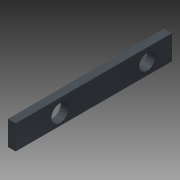
# Autodesk Inventor part: connector
Saved by Autodesk Inventor 2015 (Build 190159000, 159)
## iProperties
Created: 2020-01-20
Part Number: connector
Material: Iron, Cast
Document SubType Name: Modeling
Designer: hp
Density: 7.15 g/cm^3
Appearance: Iron Gray
Author: hp
Autodesk Inventor part; units mm, degrees
ref_plane "YZ Plane" through (0, 0, 0) normal (1, 0, 0) x (0, 1, 0)
ref_plane "XZ Plane" through (0, 0, 0) normal (0, 1, 0) x (-1, 0, 0)
ref_plane "XY Plane" through (0, 0, 0) normal (0, 0, 1) x (1, 0, 0)
sketch "Sketch1" plane through (0, 0, 0) normal (1, 0, 0) x (0, 1, 0)
  line L0 (-28.0063, 19.8873) -> (-28.0062, -488.1127)
  line L1 (-106.9702, 19.8873) -> (-28.0063, 19.8873)
  circle A0 centre (-68.4003, -407.0636) radius 25.4
  line L2 (-106.9702, -488.1127) -> (-28.0062, -488.1127)
  line L3 (-106.9702, -488.1127) -> (-106.9702, 19.8873)
  line L4 (-68.4003, -407.0636) -> (-65.1463, -90.9011)
  circle A1 centre (-65.1463, -90.9011) radius 25.4
  point P0 (0, 0)
  dimension "d0" = 508
  dimension "d2" = 50.8
  dimension "d5" = 316.1792
  dimension "d6" = 50.8
  constraints: 10 end point, 2 centre point, 1 coincident, 1 horizontal, 1 perpendicular, 1 vertical
  measures "d0" distance of L0.start L0.end
  measures "d2" diameter of A0
  measures "d5" distance of L4.start L4.end
  measures "d6" diameter of A1
extrude "Extrusion1" add sketch "Sketch1" along normal blind 25.4 contours L0 L2 L3 L1 | A1
sketch "Sketch2" plane through (25.4, 0, 0) normal (1, 0, 0) x (0, 0, -1)
  circle A0 centre (407.0405, -68.16) radius 25.3847
  line L0 (407.0405, -70.7875) -> (123.9383, -70.7875)
  circle A1 centre (123.9383, -70.7875) radius 27.94
  point P0 (0, 0)
  dimension "d7" = 283.1022
  dimension "d8" = 55.88
  constraints: 2 centre point, 2 end point, 1 coincident, 1 horizontal
  measures "d7" distance of L0.start L0.end
  measures "d8" diameter of A1
extrude "Extrusion2" cut sketch "Sketch2" against normal blind 25.4 contours A1
body "Solid1"
